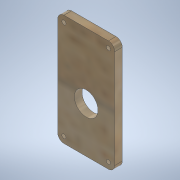
# Autodesk Inventor part: 上下直動t5.5_エンコーダ軸受け
Saved by Autodesk Inventor 2020.3 (Build 243373000, 373)
## iProperties
Created: 2020-07-07
Part Number: 上下直動t5.5_エンコーダ軸受け
Material: 木材 (カエデ材)
Document SubType Name: Modeling
Designer: totot
Density: 0.67 g/cm^3
Appearance: ナチュラル カエデ材 - 光沢 濃い着色
Author: totot
Autodesk Inventor part; units mm, degrees
ref_plane "YZ Plane" through (0, 0, 0) normal (1, 0, 0) x (0, 1, 0)
ref_plane "XZ Plane" through (0, 0, 0) normal (0, 1, 0) x (-1, 0, 0)
ref_plane "XY Plane" through (0, 0, 0) normal (0, 0, 1) x (1, 0, 0)
sketch "スケッチ1" plane through (0, 0, 0) normal (0, 0, 1) x (1, 0, 0)
  line L0 (0, 0) -> (41, 0)
  line L1 (41, 0) -> (41, -80)
  line L2 (41, -80) -> (0, -80)
  line L3 (0, -80) -> (0, 0)
  dimension "d0" = 41
  dimension "d13" = 80
  constraints: 8 end point, 2 parallel, 1 horizontal, 1 perpendicular
  measures "d0" distance of L1.end L2.end
  measures "d13" distance between parallel lines of L2 L0
extrude "押し出し1" add sketch "スケッチ1" along normal blind 5.5
sketch "スケッチ2" plane through (0, 0, 5.5) normal (0, 0, 1) x (1, 0, 0)
  line L0 (4.5, -75.5) -> (36.5, -75.5)
  line L1 (36.5, -75.5) -> (36.5, -4.5)
  line L2 (36.5, -4.5) -> (4.5, -4.5)
  line L3 (4.5, -4.5) -> (4.5, -75.5)
  line L4 (0, -80) -> (41, -80) projected
  line L5 (0, 0) -> (0, -80) projected
  dimension "d3" = 4.5
  dimension "d4" = 32
  dimension "d5" = 4.5
  dimension "d14" = 71
  constraints: 8 end point, 4 coincident, 2 parallel, 1 horizontal, 1 perpendicular
  measures "d3" distance between parallel lines of L4 L0
  measures "d4" distance of L1.end L2.end
  measures "d5" distance between parallel lines of L5 L3
  measures "d14" distance of L2.end L0.start
hole "穴1" at (4.5, -4.5, 5.5) at (36.5, -4.5, 5.5) at (36.5, -75.5, 5.5) at (4.5, -75.5, 5.5) direction (0, 0, -1) diameter 3 end through all
fillet "フィレット1" radius 4.5 4 edges at (0, 0, 2.75) (41, 0, 2.75) (0, -80, 2.75) (41, -80, 2.75)
sketch "スケッチ3" plane through (0, 0, 0) normal (0, 0, -1) x (-1, 0, 0)
  line L0 (-36.5, 0) -> (-4.5, 0) projected
  line L1 (0, -4.5) -> (0, -75.5) projected
  line L2 (-41, -75.5) -> (-41, -4.5) projected
  point P0 (0, 0)
  point P1 (-20.5, -47)
  dimension "d16" = 47
  dimension "d17" = 41
  dimension "d18" = 20.5
  measures "d16" distance from line of point (-20.5, -47) L0
  measures "d17" distance between parallel lines of L1 L2
  measures "d18" distance from line of point (-20.5, -47) L2
hole "穴2" at (20.5, -47, 0) direction (0, 0, 1) diameter 17 end through all
sketch "スケッチ4" plane through (0, 0, 0) normal (0, 0, -1) x (-1, 0, 0)
  line L0 (0, -4.5) -> (0, -75.5) projected
  line L1 (-36.5, 0) -> (-4.5, 0) projected
  line L2 (-4.5, -80) -> (-36.5, -80) projected
  point P0 (0, 0)
  point P1 (-5.5, -10)
  point P2 (-5.5, -15)
  point P3 (-5.5, -20)
  point P4 (-5.5, -25)
  point P5 (-5.5, -30)
  point P6 (-5.5, -35)
  point P7 (-10.5, -10)
  point P8 (-10.5, -15)
  point P9 (-10.5, -20)
  point P10 (-10.5, -25)
  point P11 (-10.5, -30)
  point P12 (-10.5, -35)
  point P13 (-15.5, -10)
  point P14 (-15.5, -15)
  point P15 (-15.5, -20)
  point P16 (-15.5, -25)
  point P17 (-15.5, -30)
  point P18 (-15.5, -35)
  point P19 (-20.5, -10)
  point P20 (-20.5, -15)
  point P21 (-20.5, -20)
  point P22 (-20.5, -25)
  point P23 (-20.5, -30)
  point P24 (-20.5, -35)
  point P25 (-25.5, -10)
  point P26 (-25.5, -15)
  point P27 (-25.5, -20)
  point P28 (-25.5, -25)
  point P29 (-25.5, -30)
  point P30 (-25.5, -35)
  point P31 (-30.5, -10)
  point P32 (-30.5, -15)
  point P33 (-30.5, -20)
  point P34 (-30.5, -25)
  point P35 (-30.5, -30)
  point P36 (-30.5, -35)
  point P37 (-35.5, -10)
  point P38 (-35.5, -15)
  point P39 (-35.5, -20)
  point P40 (-35.5, -25)
  point P41 (-35.5, -30)
  point P42 (-35.5, -35)
  point P43 (-5.5, -70)
  point P44 (-5.5, -65)
  point P45 (-5.5, -60)
  point P46 (-10.5, -70)
  point P47 (-10.5, -65)
  point P48 (-10.5, -60)
  point P49 (-15.5, -70)
  point P50 (-15.5, -65)
  point P51 (-15.5, -60)
  point P52 (-20.5, -70)
  point P53 (-20.5, -65)
  point P54 (-20.5, -60)
  point P55 (-25.5, -70)
  point P56 (-25.5, -65)
  point P57 (-25.5, -60)
  point P58 (-30.5, -70)
  point P59 (-30.5, -65)
  point P60 (-30.5, -60)
  point P61 (-35.5, -70)
  point P62 (-35.5, -65)
  point P63 (-35.5, -60)
  dimension "d26" = 5.5
  dimension "d27" = 10
  dimension "d30" = 5
  dimension "d33" = 5
  dimension "d36" = 5.5
  dimension "d37" = 10
  dimension "d40" = 5
  dimension "d43" = 5
  constraints: 2 horizontal, 2 vertical, 61 other
  measures "d26" distance from line of point (-5.5, -10) L0
  measures "d27" distance from line of point (-5.5, -10) L1
  measures "d30" distance of point (-5.5, -10) point (-5.5, -15)
  measures "d33" distance of point (-5.5, -10) point (-10.5, -10)
  measures "d36" distance from line of point (-5.5, -70) L0
  measures "d37" distance from line of point (-5.5, -70) L2
  measures "d40" distance of point (-5.5, -70) point (-5.5, -65)
  measures "d43" distance of point (-5.5, -70) point (-10.5, -70)
hole "穴3" at (5.5, -10, 0) at (5.5, -15, 0) at (5.5, -20, 0) at (5.5, -25, 0) at (5.5, -30, 0) at (5.5, -35, 0) at (10.5, -10, 0) at (10.5, -15, 0) at (10.5, -20, 0) at (10.5, -25, 0) at (10.5, -30, 0) at (10.5, -35, 0) at (15.5, -10, 0) at (15.5, -15, 0) at (15.5, -20, 0) at (15.5, -25, 0) at (15.5, -30, 0) at (15.5, -35, 0) at (20.5, -10, 0) at (20.5, -15, 0) at (20.5, -20, 0) at (20.5, -25, 0) at (20.5, -30, 0) at (20.5, -35, 0) at (25.5, -10, 0) at (25.5, -15, 0) at (25.5, -20, 0) at (25.5, -25, 0) at (25.5, -30, 0) at (25.5, -35, 0) at (30.5, -10, 0) at (30.5, -15, 0) at (30.5, -20, 0) at (30.5, -25, 0) at (30.5, -30, 0) at (30.5, -35, 0) at (35.5, -10, 0) at (35.5, -15, 0) at (35.5, -20, 0) at (35.5, -25, 0) at (35.5, -30, 0) at (35.5, -35, 0) at (5.5, -70, 0) at (5.5, -65, 0) at (5.5, -60, 0) at (10.5, -70, 0) at (10.5, -65, 0) at (10.5, -60, 0) at (15.5, -70, 0) at (15.5, -65, 0) direction (0, 0, 1) diameter 3.5 end through all and at (15.5, -60, 0) (20.5, -70, 0) (20.5, -65, 0) (20.5, -60, 0) (25.5, -70, 0) (25.5, -65, 0) (25.5, -60, 0) (30.5, -70, 0) (30.5, -65, 0) (30.5, -60, 0) (35.5, -70, 0) (35.5, -65, 0) (35.5, -60, 0)
equation "\"d18\" = 0.5 * d17"
equation "\"d36\" = d26"
